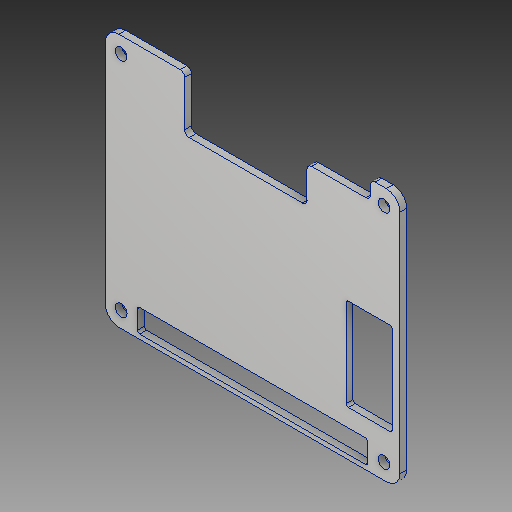
# Autodesk Inventor part: ボードガード
Saved by Autodesk Inventor 2017 (Build 210142000, 142)
## iProperties
Created: 2016-10-31
Part Number: ボードガード
Material: アルミニウム 6061
Document SubType Name: Modeling
Designer: NN
Mass: 11.2062 g
Surface Area: 62.2683 cm^2
Volume: 4.15043 cm^3
Density: 2.7 g/cm^3
Appearance: アルミニウム - フラット
Author: NN
Autodesk Inventor part; units mm, degrees
ref_plane "YZ Plane" through (0, 0, 0) normal (1, 0, 0) x (0, 1, 0)
ref_plane "XZ Plane" through (0, 0, 0) normal (0, 1, 0) x (-1, 0, 0)
ref_plane "XY Plane" through (0, 0, 0) normal (0, 0, 1) x (1, 0, 0)
sketch "スケッチ1" plane through (0, 0, 0) normal (0, 0, 1) x (1, 0, 0)
  line L0 (0, 0) -> (65, 0)
  line L1 (65, 0) -> (65, 56)
  line L2 (65, 56) -> (0, 56)
  line L3 (0, 56) -> (0, 0)
  dimension "d0" = 56
  dimension "d1" = 65
  constraints: 8 end point, 2 parallel, 1 horizontal, 1 perpendicular
  measures "d0" distance of L2.end L0.start
  measures "d1" distance of L0.start L0.end
extrude "押し出し1" add sketch "スケッチ1" along normal blind 1.5
sketch "スケッチ2" plane through (0, 0, 1.5) normal (0, 0, 1) x (1, 0, 0)
  line L0 (0, 0) -> (65, 0) projected
  line L1 (65, 0) -> (65, 56) projected
  line L2 (65, 56) -> (0, 56) projected
  line L3 (0, 56) -> (0, 0) projected
  line L4 (3.5, 52.5) -> (61.5, 52.5)
  line L5 (61.5, 52.5) -> (61.5, 3.5)
  line L6 (61.5, 3.5) -> (3.5, 3.5)
  line L7 (3.5, 3.5) -> (3.5, 52.5)
  dimension "d4" = 3.5
  constraints: 8 end point, 3 other
  measures "d4" distance between parallel lines of L7 L3
hole "穴1" at (61.5, 52.5, 1.5) at (61.5, 3.5, 1.5) at (3.5, 3.5, 1.5) at (3.5, 52.5, 1.5) direction (0, 0, -1) diameter 2.6 end through all
fillet "フィレット1" radius 3 4 edges at (0, 56, 0.75) (65, 56, 0.75) (65, 0, 0.75) (0, 0, 0.75)
sketch "スケッチ3" plane through (0, 0, 1.5) normal (0, 0, 1) x (1, 0, 0)
  arc A0 (0, 3) -> (3, 0) centre (3, 3) ccw projected
  line L0 (3, 0) -> (62, 0) projected
  arc A1 (62, 0) -> (65, 3) centre (62, 3) ccw projected
  line L1 (65, 3) -> (65, 53) projected
  arc A2 (65, 53) -> (62, 56) centre (62, 53) ccw projected
  line L2 (62, 56) -> (3, 56) projected
  arc A3 (3, 56) -> (0, 53) centre (3, 53) ccw projected
  line L3 (0, 53) -> (0, 3) projected
  circle A4 centre (3.5, 3.5) radius 1.3 projected
  circle A5 centre (61.5, 52.5) radius 1.3 projected
  circle A6 centre (61.5, 3.5) radius 1.3 projected
  circle A7 centre (3.5, 52.5) radius 1.3 projected
  line L4 (63.3, 30.32) -> (53.14, 30.32)
  line L5 (53.14, 30.32) -> (53.14, 10)
  line L6 (53.14, 10) -> (63.3, 10)
  line L7 (63.3, 10) -> (63.3, 30.32)
  point P0 (0, 0)
  dimension "d13" = 20.32
  dimension "d14" = 10.16
  dimension "d23" = 1.7
  dimension "d24" = 10
  constraints: 8 end point, 2 parallel, 1 horizontal, 1 perpendicular
  measures "d13" distance of L6.end L4.start
  measures "d14" distance of L5.end L6.end
  measures "d23" distance between parallel lines of L1 L7
  measures "d24" distance between parallel lines of L0 L6
extrude "押し出し2" cut sketch "スケッチ3" against normal through all contours L7 L6 L5 L4
sketch "スケッチ4" plane through (0, 0, 1.5) normal (0, 0, 1) x (1, 0, 0)
  line L0 (53.14, 10) -> (53.14, 30.32) projected
  line L1 (53.14, 30.32) -> (63.3, 30.32) projected
  line L2 (63.3, 30.32) -> (63.3, 10) projected
  line L3 (63.3, 10) -> (53.14, 10) projected
  arc A0 (0, 3) -> (3, 0) centre (3, 3) ccw projected
  line L4 (3, 0) -> (62, 0) projected
  arc A1 (62, 0) -> (65, 3) centre (62, 3) ccw projected
  line L5 (65, 3) -> (65, 53) projected
  arc A2 (65, 53) -> (62, 56) centre (62, 53) ccw projected
  line L6 (62, 56) -> (3, 56) projected
  arc A3 (3, 56) -> (0, 53) centre (3, 53) ccw projected
  line L7 (0, 53) -> (0, 3) projected
  circle A4 centre (3.5, 3.5) radius 1.3 projected
  circle A5 centre (61.5, 52.5) radius 1.3 projected
  circle A6 centre (61.5, 3.5) radius 1.3 projected
  circle A7 centre (3.5, 52.5) radius 1.3 projected
  line L8 (57.9, 1) -> (7.1, 1)
  line L9 (7.1, 1) -> (7.1, 6.08)
  line L10 (7.1, 6.08) -> (57.9, 6.08)
  line L11 (57.9, 6.08) -> (57.9, 1)
  point P0 (0, 0)
  dimension "d17" = 5.08
  dimension "d18" = 1
  dimension "d21" = 7.1
  dimension "d22" = 50.8
  constraints: 8 end point, 2 parallel, 1 horizontal, 1 perpendicular
  measures "d17" distance of L8.end L9.end
  measures "d18" distance between parallel lines of L4 L8
  measures "d21" distance between parallel lines of L5 L11
  measures "d22" distance between parallel lines of L11 L9
extrude "押し出し3" cut sketch "スケッチ4" against normal through all contours L8 L9 L10 L11
sketch "スケッチ5" plane through (0, 0, 1.5) normal (0, 0, 1) x (1, 0, 0)
  line L0 (57.9, 6.08) -> (57.9, 1) projected
  line L1 (57.9, 1) -> (7.1, 1) projected
  line L2 (7.1, 1) -> (7.1, 6.08) projected
  line L3 (7.1, 6.08) -> (57.9, 6.08) projected
  line L4 (53.14, 10) -> (53.14, 30.32) projected
  line L5 (53.14, 30.32) -> (63.3, 30.32) projected
  line L6 (63.3, 30.32) -> (63.3, 10) projected
  line L7 (63.3, 10) -> (53.14, 10) projected
  arc A0 (0, 3) -> (3, 0) centre (3, 3) ccw projected
  line L8 (3, 0) -> (62, 0) projected
  arc A1 (62, 0) -> (65, 3) centre (62, 3) ccw projected
  line L9 (65, 3) -> (65, 53) projected
  arc A2 (65, 53) -> (62, 56) centre (62, 53) ccw projected
  line L10 (62, 56) -> (3, 56) projected
  arc A3 (3, 56) -> (0, 53) centre (3, 53) ccw projected
  line L11 (0, 53) -> (0, 3) projected
  circle A4 centre (3.5, 3.5) radius 1.3 projected
  circle A5 centre (61.5, 52.5) radius 1.3 projected
  circle A6 centre (61.5, 3.5) radius 1.3 projected
  circle A7 centre (3.5, 52.5) radius 1.3 projected
  line L12 (58.5, 56) -> (44.5, 56)
  line L13 (44.5, 56) -> (44.5, 52)
  line L14 (44.5, 52) -> (58.5, 52)
  line L15 (58.5, 52) -> (58.5, 56)
  line L16 (17.5, 44) -> (44.5, 44)
  line L17 (44.5, 44) -> (44.5, 56)
  line L18 (44.5, 56) -> (17.5, 56)
  line L19 (17.5, 56) -> (17.5, 44)
  point P0 (0, 0)
  dimension "d25" = 3
  dimension "d26" = 4
  dimension "d27" = 14
  dimension "d28" = 27
  dimension "d29" = 12
  constraints: 16 end point, 4 parallel, 2 horizontal, 2 perpendicular, 1 point on line
  measures "d25" distance from line of A5.centre L15
  measures "d26" distance between parallel lines of L12 L14
  measures "d27" distance between parallel lines of L13 L15
  measures "d28" distance between parallel lines of L19 L17
  measures "d29" distance between parallel lines of L16 L18
extrude "押し出し4" cut sketch "スケッチ5" against normal through all contours L10 L13 L17 L16 L19 | L10 L15 L14 L13
fillet "フィレット2" radius 1 3 edges at (58.5, 56, 0.75) (44.5, 52, 0.75) (17.5, 56, 0.75)
fillet "フィレット2" radius 1 3 edges at (58.5, 52, 0.75) (44.5, 44, 0.75) (17.5, 44, 0.75)
fillet "フィレット3" radius 0.5 8 edges at (57.9, 1, 0.75) (57.9, 6.08, 0.75) (63.3, 10, 0.75) (53.14, 10, 0.75) (53.14, 30.32, 0.75) (63.3, 30.32, 0.75) (7.1, 1, 0.75) (7.1, 6.08, 0.75)
